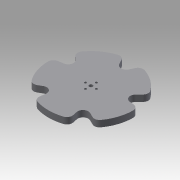
# Autodesk Inventor part: gear wheel
Saved by Autodesk Inventor 2016 (Build 200138000, 138)
## iProperties
Created: 2015-11-24
Part Number: gear wheel
Material: Generic
Document SubType Name: Modeling
Designer: Delta
Density: 1 g/cm^3
Appearance: Default
Author: Delta
Autodesk Inventor part; units mm, degrees
ref_plane "YZ Plane" through (0, 0, 0) normal (1, 0, 0) x (0, 1, 0)
ref_plane "XZ Plane" through (0, 0, 0) normal (0, 1, 0) x (-1, 0, 0)
ref_plane "XY Plane" through (0, 0, 0) normal (0, 0, 1) x (1, 0, 0)
sketch "Sketch1" plane through (0, 0, 0) normal (0, 1, 0) x (-1, 0, 0)
  circle A0 centre (0, 0) radius 76.2
  dimension "d0" = 152.4
  constraints: 2 coincident, 1 centre point
  measures "d0" diameter of A0
extrude "Extrusion1" add sketch "Sketch1" along normal blind 11.43
sketch "Sketch2" plane through (0, 11.43, 0) normal (0, 1, 0) x (1, 0, 0)
  circle A0 centre (0, 0) radius 76.2 projected
  line L0 (0.1023, 76.1999) -> (0.1023, 63.4999) construction
  arc A1 (-8.3552, 59.1187) -> (8.4222, 58.8626) centre (0.1023, 63.4999) ccw
  line L1 (8.4222, 58.8626) -> (15.4584, 74.6155)
  line L2 (-8.3552, 59.1187) -> (-16.2911, 74.4382)
  dimension "d3" = 12.7
  dimension "d4" = 19.05
  dimension "d16" = 31.75
  constraints: 6 end point, 5 point on circle, 1 centre point, 1 coincident, 1 equal length, 1 tangent, 1 vertical
  measures "d3" distance of L0.start L0.end
  measures "d4" diameter of A1
  measures "d16" distance of L2.end L1.end
extrude "Extrusion2" cut sketch "Sketch2" against normal through all contours L1 A1 L2 A0 picked at (1.6562, 64.6745)
fillet "Fillet1" radius 9.525 1 edges at (-16.2911, 5.715, -74.4382)
fillet "Fillet2" radius 9.525 1 edges at (15.4584, 5.715, -74.6155)
pattern_circular "Circular Pattern1" count 5 over 360 about axis through (0, -10, 0) along (0, 1, 0) of "Extrusion2", "Fillet1", "Fillet2"
sketch "Sketch4" plane through (0, 0, 0) normal (0, -1, 0) x (1, 0, 0)
  circle A0 centre (0, 0) radius 3.175
  dimension "d19" = 6.35
  constraints: 1 centre point, 1 coincident
  measures "d19" diameter of A0
hole "Hole1" at (0, 0, 0) direction (0, 1, 0) diameter 6.35 end through all
sketch "Sketch5" plane through (0, 0, 0) normal (0, -1, 0) x (1, 0, 0)
  circle A0 centre (0, -9.779) radius 1.9844
  circle A1 centre (0, 0) radius 3.175 projected
  arc A2 (67.6814, -9.2124) -> (76.1994, 0.2962) centre (66.6745, 0.2592) ccw projected
  arc A3 (76.1994, 0.2962) -> (62.0688, 44.203) centre (0, 0) ccw projected
  arc A4 (62.0688, 44.203) -> (50.0431, 47.1934) centre (54.3102, 38.6777) ccw projected
  line L0 (50.0431, 47.1934) -> (41.5086, 42.9169) projected
  arc A5 (27.7848, 52.5712) -> (41.5086, 42.9169) centre (37.2415, 51.4327) ccw projected
  line L1 (27.7848, 52.5712) -> (29.6763, 61.522) projected
  arc A6 (29.6763, 61.522) -> (23.2652, 72.5615) centre (20.357, 63.4913) ccw projected
  arc A7 (23.2652, 72.5615) -> (-22.8593, 72.6904) centre (0, 0) ccw projected
  arc A8 (-22.8593, 72.6904) -> (-29.4194, 62.1774) centre (-20.0019, 63.6041) ccw projected
  line L2 (-29.4194, 62.1774) -> (-27.9896, 52.7391) projected
  arc A9 (-41.4122, 42.6704) -> (-27.9896, 52.7391) centre (-37.4071, 51.3124) ccw projected
  line L3 (-41.4122, 42.6704) -> (-49.3405, 47.2352) projected
  arc A10 (-49.3405, 47.2352) -> (-61.8207, 44.5493) centre (-54.0931, 38.9806) ccw projected
  arc A11 (-61.8207, 44.5493) -> (-76.1966, 0.7221) centre (0, 0) ccw projected
  arc A12 (-76.1966, 0.7221) -> (-68.2253, -8.7657) centre (-66.672, 0.6318) ccw projected
  line L4 (-68.2253, -8.7657) -> (-58.8071, -10.3224) projected
  arc A13 (-53.379, -26.1995) -> (-58.8071, -10.3224) centre (-60.3604, -19.7199) ccw projected
  line L5 (-53.379, -26.1995) -> (-60.1703, -32.3291) projected
  arc A14 (-60.1703, -32.3291) -> (-61.4725, -45.0285) centre (-53.7885, -39.4) ccw projected
  arc A15 (-61.4725, -45.0285) -> (-24.2328, -72.2441) centre (0, 0) ccw projected
  arc A16 (-24.2328, -72.2441) -> (-12.7461, -67.5948) centre (-21.2037, -63.2136) ccw projected
  line L6 (-12.7461, -67.5948) -> (-8.3552, -59.1187) projected
  arc A17 (8.4222, -58.8626) -> (-8.3552, -59.1187) centre (0.1023, -63.4999) ccw projected
  line L7 (8.4222, -58.8626) -> (12.1532, -67.2156) projected
  arc A18 (12.1532, -67.2156) -> (23.8286, -72.3784) centre (20.8501, -63.3311) ccw projected
  arc A19 (23.8286, -72.3784) -> (61.2199, -45.3714) centre (0, 0) ccw projected
  arc A20 (61.2199, -45.3714) -> (60.3477, -33.0102) centre (53.5674, -39.7) ccw projected
  line L8 (60.3477, -33.0102) -> (53.6433, -26.215) projected
  arc A21 (58.5842, -10.1795) -> (53.6433, -26.215) centre (60.4236, -19.5253) ccw projected
  line L9 (58.5842, -10.1795) -> (67.6814, -9.2124) projected
  circle A22 centre (0, 0) radius 3.175 projected
  circle A23 centre (0, 0) radius 3.175 projected
  circle A24 centre (0, 0) radius 3.175 projected
  circle A25 centre (9.779, 0) radius 1.9844
  circle A26 centre (0, 9.779) radius 1.9844
  circle A27 centre (-9.779, 0) radius 1.9844
  dimension "d27" = 9.779
  dimension "d28" = 3.9688
  dimension "d31" = 360
  constraints: 4 centre point, 2 coincident, 11 other
  measures "d27" distance of A0.centre point (0, 0)
  measures "d28" diameter of A0
extrude "Extrusion3" cut sketch "Sketch5" against normal blind 12.7 contours A0 | A25 | A26 | A27
body "Solid1"
